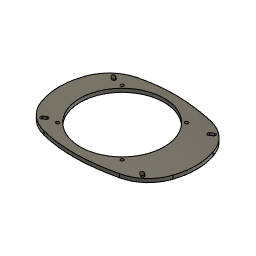
6x9_speaker_adapter_ v1 (Autodesk Fusion 360 design; units mm, degrees)
Autodesk Fusion 360 part; units mm, degrees
sketch "Sketch1" plane through (0, 0, 0) normal (0, 1, 0) x (1, 0, 0)
  circle A0 centre (0, 0) radius 71.65
  circle A1 centre (0, 0) radius 83.65
  circle A2 centre (0, 0) radius 86.15 construction
  line L0 (0, 0) -> (10, 0) construction
  line L1 (-106.5, 0) -> (126.5, 0) construction
  line L2 (-84.5, -69.5) -> (104.5, -69.5) construction
  line L3 (104.5, -69.5) -> (104.5, 69.5) construction
  line L4 (104.5, 69.5) -> (-84.5, 69.5) construction
  line L5 (-84.5, 69.5) -> (-84.5, -69.5) construction
  line L6 (-84.5, -69.5) -> (104.5, 69.5) construction
  line L7 (104.5, -69.5) -> (-84.5, 69.5) construction
  line L8 (93.5, -59) -> (-73.5, -59) construction
  line L9 (-73.5, -59) -> (-73.5, 59) construction
  line L10 (-73.5, 59) -> (93.5, 59) construction
  line L11 (93.5, 59) -> (93.5, -59) construction
  line L12 (93.5, -59) -> (-73.5, 59) construction
  line L13 (-73.5, -59) -> (93.5, 59) construction
  line L14 (0, 86.15) -> (0, -86.15) construction
  circle A3 centre (0, 0) radius 77.65 construction
  line L15 (0, 0) -> (54.9068, -54.9068) construction
  line L16 (0, 0) -> (77.65, 0) construction
  point P0 (10, 0)
  point P1 (10, 0)
  dimension "d1" = 143.3
  dimension "d2" = 167.3
  dimension "d3" = 172.3
  dimension "d5" = 10
  dimension "d6" = 233
  dimension "d7" = 189
  dimension "d8" = 139
  dimension "d9" = 167
  dimension "d10" = 118
  dimension "d22" = 155.3
  dimension "d23" = 45
  constraint coincident A0.centre A1.centre
  constraint concentric A1 A2
  constraint horizontal L0
  constraint parallel L0 L1
  constraint midpoint P1 L1
  constraint horizontal L2
  constraint perpendicular L2 L3
  constraint parallel L2 L4
  constraint parallel L3 L5
  constraint coincident L6 P1
  constraint coincident L7 P1
  constraint coincident P1 P0
  constraint horizontal L8
  constraint perpendicular L8 L9
  constraint parallel L8 L10
  constraint parallel L9 L11
  constraint coincident L12 P1
  constraint coincident L13 P1
  constraint coincident A2 L14.start
  constraint coincident A2 L14.end
  constraint vertical L14
  constraint concentric A1 A3
  constraint horizontal L16
  constraint coincident A3 L15.end
  measures "d1" diameter of A0
  measures "d2" diameter of A1
  measures "d3" diameter of A2
  measures "d5" distance of A0.centre P1
  measures "d6" distance of L1.start L1.end
  measures "d7" distance of L3.end L4.end
  measures "d8" distance of L2.end L3.end
  measures "d9" distance of L9.end L10.end
  measures "d10" distance of L8.end L9.end
  measures "d22" diameter of A3
  measures "d23" angle of L15 L16
sketch "Sketch2" plane through (0, 0, 0) normal (0, 1, 0) x (1, 0, 0)
  spline S0 degree 5 poles (-84.5, 69.5) (-81.1215, 70.7869) (-74.3286, 73.2455) (-64.0315, 76.5883) (-50.083, 80.3433) (-32.2585, 83.7904) (-14.0132, 85.8889) (4.6825, 86.5435) (23.8364, 85.73) (43.4214, 83.5343) (63.4013, 80.0731) (79.6732, 76.3808) (92.0287, 73.1261) (100.3319, 70.7441) (104.5, 69.5) knots 0 0 0 0 0 0 0.1 0.2 0.3 0.4 0.5 0.6 0.7 0.8 0.9 1 1 1 1 1 1
  line L0 (104.5, 69.5) -> (-84.5, 69.5)
  spline S1 degree 5 poles (-84.5, -69.5) (-81.1215, -70.7869) (-74.3286, -73.2455) (-64.0315, -76.5883) (-50.083, -80.3433) (-32.2585, -83.7904) (-14.0132, -85.8889) (4.6825, -86.5435) (23.8364, -85.73) (43.4214, -83.5343) (63.4013, -80.0731) (79.6732, -76.3808) (92.0287, -73.1261) (100.3319, -70.7441) (104.5, -69.5) knots 0 0 0 0 0 0 0.1 0.2 0.3 0.4 0.5 0.6 0.7 0.8 0.9 1 1 1 1 1 1
  line L1 (104.5, -69.5) -> (104.5, 69.5)
  spline S2 degree 5 poles (-84.5, 69.5) (-86.1686, 66.72) (-89.3602, 61.16) (-93.7104, 52.82) (-98.6219, 41.7) (-103.1794, 27.8) (-106.0136, 13.9) (-106.9839, 0) (-106.0136, -13.9) (-103.1794, -27.8) (-98.6219, -41.7) (-93.7104, -52.82) (-89.3602, -61.16) (-86.1686, -66.72) (-84.5, -69.5) knots 0 0 0 0 0 0 0.1 0.2 0.3 0.4 0.5 0.6 0.7 0.8 0.9 1 1 1 1 1 1
  spline S3 degree 5 poles (104.5, 69.5) (106.1686, 66.72) (109.3602, 61.16) (113.7104, 52.82) (118.6219, 41.7) (123.1794, 27.8) (126.0136, 13.9) (126.9839, 0) (126.0136, -13.9) (123.1794, -27.8) (118.6219, -41.7) (113.7104, -52.82) (109.3602, -61.16) (106.1686, -66.72) (104.5, -69.5) knots 0 0 0 0 0 0 0.1 0.2 0.3 0.4 0.5 0.6 0.7 0.8 0.9 1 1 1 1 1 1
  point P0 (0, 86.15)
  point P1 (-84.5, 69.5)
  point P2 (0, 86.15)
  point P3 (104.5, 69.5)
  point P4 (0, -86.15)
  point P5 (-84.5, -69.5)
  point P6 (0, -86.15)
  point P7 (104.5, -69.5)
  point P8 (-106.5, 0)
  point P9 (-106.5, 0)
  point P10 (126.5, 0)
  point P11 (126.5, 0)
  constraint coincident S0.start L0.end
  constraint coincident P0 P2
  constraint coincident S0.end L0.start
  constraint coincident P5 S1.start
  constraint coincident P6 P4
  constraint coincident P7 S1.end
  constraint coincident P9 P8
  constraint coincident P11 P10
sketch "Sketch3" plane through (0, 0, 0) normal (0, 1, 0) x (1, 0, 0)
  line L0 (-77.5372, 58.4854) -> (-72.637, 55.023)
  arc A0 (-72.637, 55.023) -> (-69.4632, 59.5149) centre (-71.0501, 57.2689) ccw
  line L1 (-69.4632, 59.5149) -> (-74.3634, 62.9773)
  arc A1 (-74.3634, 62.9773) -> (-77.5372, 58.4854) centre (-75.9503, 60.7313) ccw
  line L2 (-75.9503, 60.7313) -> (-71.0501, 57.2689) construction
  line L3 (93.5, -59) -> (-73.5, 59)
  line L4 (-73.5, -59) -> (93.5, 59)
  line L5 (94.3632, 62.9771) -> (89.463, 59.5147)
  arc A2 (89.463, 59.5147) -> (92.6368, 55.0229) centre (91.0499, 57.2688) ccw
  line L6 (92.6368, 55.0229) -> (97.537, 58.4853)
  arc A3 (97.537, 58.4853) -> (94.3632, 62.9771) centre (95.9501, 60.7312) ccw
  line L7 (95.9501, 60.7312) -> (91.0499, 57.2688) construction
  line L8 (97.537, -58.4853) -> (92.6368, -55.0229)
  arc A4 (92.6368, -55.0229) -> (89.463, -59.5147) centre (91.0499, -57.2688) ccw
  line L9 (89.463, -59.5147) -> (94.3632, -62.9771)
  arc A5 (94.3632, -62.9771) -> (97.537, -58.4853) centre (95.9501, -60.7312) ccw
  line L10 (95.9501, -60.7312) -> (91.0499, -57.2688) construction
  line L11 (-74.3632, -62.9771) -> (-69.463, -59.5147)
  arc A6 (-69.463, -59.5147) -> (-72.6368, -55.0229) centre (-71.0499, -57.2688) ccw
  line L12 (-72.6368, -55.0229) -> (-77.537, -58.4853)
  arc A7 (-77.537, -58.4853) -> (-74.3632, -62.9771) centre (-75.9501, -60.7312) ccw
  line L13 (-75.9501, -60.7312) -> (-71.0499, -57.2688) construction
  line L14 (-80.541, 57.6998) -> (-72.374, 51.9291)
  arc A8 (-72.374, 51.9291) -> (-66.459, 60.3002) centre (-69.4165, 56.1147) ccw
  line L15 (-66.459, 60.3002) -> (-74.626, 66.0709)
  arc A9 (-74.626, 66.0709) -> (-80.541, 57.6998) centre (-77.5835, 61.8853) ccw
  line L16 (-77.5835, 61.8853) -> (-69.4165, 56.1147) construction
  line L17 (94.571, 66.032) -> (86.404, 60.2613)
  arc A10 (86.404, 60.2613) -> (92.3189, 51.8902) centre (89.3615, 56.0758) ccw
  line L18 (92.3189, 51.8902) -> (100.4859, 57.6609)
  arc A11 (100.4859, 57.6609) -> (94.571, 66.032) centre (97.5284, 61.8464) ccw
  line L19 (97.5284, 61.8464) -> (89.3615, 56.0758) construction
  line L20 (100.541, -57.6998) -> (92.374, -51.9291)
  arc A12 (92.374, -51.9291) -> (86.459, -60.3002) centre (89.4165, -56.1147) ccw
  line L21 (86.459, -60.3002) -> (94.626, -66.0709)
  arc A13 (94.626, -66.0709) -> (100.541, -57.6998) centre (97.5835, -61.8853) ccw
  line L22 (97.5835, -61.8853) -> (89.4165, -56.1147) construction
  line L23 (-74.626, -66.0709) -> (-66.459, -60.3002)
  arc A14 (-66.459, -60.3002) -> (-72.374, -51.9291) centre (-69.4165, -56.1147) ccw
  line L24 (-72.374, -51.9291) -> (-80.541, -57.6998)
  arc A15 (-80.541, -57.6998) -> (-74.626, -66.0709) centre (-77.5835, -61.8853) ccw
  line L25 (-77.5835, -61.8853) -> (-69.4165, -56.1147) construction
  point P0 (-73.5002, 59.0001)
  point P1 (93.5, 59)
  point P2 (93.5, -59)
  point P3 (-73.5, -59)
  point P4 (-73.5, 59)
  point P5 (93.4449, 58.9611)
  point P6 (93.5, -59)
  point P7 (-73.5, -59)
  dimension "d12" = 3
  dimension "d13" = 5.5
  dimension "d16" = 5.5
  dimension "d17" = 3
  dimension "d18" = 3
  dimension "d19" = 5.5
  dimension "d20" = 3
  dimension "d21" = 5.5
  dimension "d30" = 10.25
  dimension "d31" = 10.25
  dimension "d32" = 10.25
  dimension "d33" = 10.25
  constraint tangent L0 A0
  constraint tangent A0 L1
  constraint parallel L0 L1
  constraint tangent L1 A1
  constraint tangent L0 A1
  constraint midpoint L2 P0
  constraint parallel L1 L3
  constraint tangent L5 A2
  constraint tangent A2 L6
  constraint parallel L5 L6
  constraint tangent L6 A3
  constraint tangent L5 A3
  constraint coincident L4 A2.centre
  constraint coincident P1 L4.end
  constraint midpoint L7 P1
  constraint tangent L8 A4
  constraint tangent A4 L9
  constraint parallel L8 L9
  constraint tangent L9 A5
  constraint tangent L8 A5
  constraint coincident L3 A4.centre
  constraint coincident P6 P2
  constraint midpoint L10 P6
  constraint tangent L11 A6
  constraint tangent A6 L12
  constraint parallel L11 L12
  constraint tangent L12 A7
  constraint tangent L11 A7
  constraint coincident L4 A6.centre
  constraint parallel L4 L13
  constraint coincident P7 P3
  constraint midpoint L13 P7
  constraint tangent L14 A8
  constraint tangent A8 L15
  constraint parallel L14 L15
  constraint tangent L15 A9
  constraint tangent L14 A9
  constraint parallel L3 L16
  constraint coincident P4 L3.end
  constraint midpoint L16 P4
  constraint tangent L17 A10
  constraint tangent A10 L18
  constraint parallel L17 L18
  constraint tangent L18 A11
  constraint tangent L17 A11
  constraint parallel L4 L19
  constraint coincident L7 P5
  constraint midpoint L19 P5
  constraint tangent L20 A12
  constraint tangent A12 L21
  constraint parallel L20 L21
  constraint tangent L21 A13
  constraint tangent L20 A13
  constraint parallel L3 L22
  constraint midpoint L22 P6
  constraint tangent L23 A14
  constraint tangent A14 L24
  constraint parallel L23 L24
  constraint tangent L24 A15
  constraint tangent L23 A15
  constraint parallel L4 L25
  constraint midpoint L25 P7
  measures "d12" distance of A0.centre P0
  measures "d13" diameter of A0
  measures "d16" diameter of A2
  measures "d17" distance of A2.centre P1
  measures "d18" distance of A4.centre P6
  measures "d19" diameter of A4
  measures "d20" distance of A6.centre P7
  measures "d21" diameter of A6
  measures "d30" diameter of A8
  measures "d31" diameter of A10
  measures "d32" diameter of A12
  measures "d33" diameter of A14
sketch "Sketch4" plane through (0, 0, 0) normal (0, 1, 0) x (1, 0, 0)
  circle A0 centre (54.9068, -54.9068) radius 2.625
  circle A1 centre (54.9068, -54.9068) radius 6
  circle A2 centre (54.9068, 54.9068) radius 2.625
  circle A3 centre (54.9068, 54.9068) radius 6
  circle A4 centre (-54.9068, 54.9068) radius 2.625
  circle A5 centre (-54.9068, 54.9068) radius 6
  circle A6 centre (-54.9068, -54.9068) radius 2.625
  circle A7 centre (-54.9068, -54.9068) radius 6
  point P0 (54.9068, -54.9068)
  dimension "d24" = 5.25
  dimension "d25" = 12
  dimension "d27" = 360
  constraint coincident P0 A0.centre
  measures "d24" diameter of A0
  measures "d25" diameter of A1
extrude "Extrude1" add sketch "Sketch2" against normal blind 6
extrude "Extrude4" cut sketch "Sketch3" sketch "Sketch4" sketch "Sketch1" along normal up to surface contours L0 A0 L1 A1 | L5 A2 L6 A3 | L8 A4 L9 A5 | L11 A6 L12 A7 of sketch 2 contours A0 | A2 | A4 | A6 of sketch 3 contours A0 end surface through (0, -6, 0) normal (0, 1, 0) offset 0
fillet "Fillet2" radius 65 4 edges at (104.5, -3, 69.5) (104.5, -3, -69.5) (-84.5, -3, 69.5) (-84.5, -3, -69.5)
